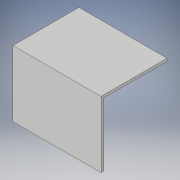
# Autodesk Inventor part: corner piece 2x1.5
Saved by Autodesk Inventor 2017 (Build 210142000, 142)
## iProperties
Created: 2017-03-15
Part Number: corner piece 2x1.5
Material: Generic
Document SubType Name: Modeling
Designer: Jess
Density: 1 g/cm^3
Appearance: Default
Author: Jess
Autodesk Inventor part; units mm, degrees
ref_plane "YZ Plane" through (0, 0, 0) normal (1, 0, 0) x (0, 1, 0)
ref_plane "XZ Plane" through (0, 0, 0) normal (0, 1, 0) x (-1, 0, 0)
ref_plane "XY Plane" through (0, 0, 0) normal (0, 0, 1) x (1, 0, 0)
sketch "Sketch1" plane through (0, 0, 0) normal (1, 0, 0) x (0, 1, 0)
  line L0 (-16.9111, 13.1902) -> (21.1889, 13.1902)
  line L1 (21.1889, 13.1902) -> (21.1889, -24.9098)
  line L2 (21.1889, -24.9098) -> (19.6014, -24.9098)
  line L3 (19.6014, -24.9098) -> (19.6014, 11.6027)
  line L4 (19.6014, 11.6027) -> (-16.9111, 11.6027)
  line L5 (-16.9111, 11.6027) -> (-16.9111, 13.1902)
  point P0 (0, 0)
  dimension "d0" = 38.1
  dimension "d1" = 38.1
  dimension "d2" = 1.5875
  dimension "d3" = 36.5125
  dimension "d4" = 36.5125
  constraints: 12 end point, 4 perpendicular, 1 horizontal
  measures "d0" distance of L0.start L0.end
  measures "d1" distance of L0.end L1.end
  measures "d2" distance of L1.end L2.end
  measures "d3" distance of L2.end L3.end
  measures "d4" distance of L3.end L4.end
extrude "Extrusion1" add sketch "Sketch1" along normal blind 50.8
body "Solid1"
